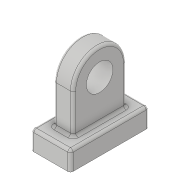
# Autodesk Inventor part: Pivot
Saved by Autodesk Inventor 2017 (Build 210142000, 142)
## iProperties
Created: 2016-07-28
Part Number: Pivot
Material: Generic
Document SubType Name: Modeling
Designer: Tutorial Books
Density: 1 g/cm^3
Appearance: Default
Author: Tutorial Books
Autodesk Inventor part; units mm, degrees
ref_plane "YZ Plane" through (0, 0, 0) normal (1, 0, 0) x (0, 1, 0)
ref_plane "XZ Plane" through (0, 0, 0) normal (0, 1, 0) x (-1, 0, 0)
ref_plane "XY Plane" through (0, 0, 0) normal (0, 0, 1) x (1, 0, 0)
sketch "Sketch1" plane through (0, 0, 0) normal (0, 1, 0) x (-1, 0, 0)
  line L0 (7.493, 14.986) -> (-7.493, 14.986)
  line L1 (-7.493, 14.986) -> (-7.493, -14.986)
  line L2 (-7.493, -14.986) -> (7.493, -14.986)
  line L3 (7.493, -14.986) -> (7.493, 14.986)
  line L4 (7.493, 14.986) -> (-7.493, -14.986) construction
  line L5 (-7.493, 14.986) -> (7.493, -14.986) construction
  point P0 (0, 0)
  dimension "d0" = 29.972
  dimension "d1" = 14.986
  constraints: 12 end point, 2 midpoint, 2 parallel, 1 horizontal, 1 perpendicular
  measures "d0" distance of L0.end L1.end
  measures "d1" distance of L1.end L2.end
extrude "Extrusion1" add sketch "Sketch1" along normal blind 7.366
sketch "Sketch2" plane through (0, 0, 0) normal (1, 0, 0) x (0, 1, 0)
  line L0 (7.366, 14.986) -> (7.366, -14.986) projected
  line L1 (7.366, 10.16) -> (22.352, 10.16)
  arc A0 (22.352, -10.16) -> (22.352, 10.16) centre (22.352, 0) ccw
  line L2 (22.352, -10.16) -> (7.366, -10.16)
  line L3 (7.366, 10.16) -> (7.366, -10.16)
  circle A1 centre (22.352, 0) radius 5.08
  point P0 (0, 0)
  dimension "d4" = 14.986
  dimension "d5" = 10.16
  dimension "d6" = 10.16
  dimension "d7" = 10.16
  constraints: 6 end point, 2 centre point, 2 point on circle, 2 point on line, 2 tangent, 1 coincident, 1 collinear, 1 horizontal, 1 parallel
  measures "d4" distance from line of L0 A0.centre
  measures "d5" radius of A0
  measures "d6" diameter of A1
  measures "d7" distance from line of L1 point (0, 0)
extrude "Extrusion2" add sketch "Sketch2" along normal mid plane 7.366
fillet "Fillet1" radius 1.016 7 edges at (7.493, 3.683, 14.986) (7.493, 7.366, 0) (7.493, 3.683, -14.986) (0, 7.366, -14.986) (0, 7.366, 14.986) (-7.493, 3.683, 14.986) (-7.493, 7.366, 0)
fillet "Fillet2" radius 1.016 6 edges at (3.683, 32.512, 0) (3.683, 14.859, -10.16) (3.683, 14.859, 10.16) (-3.683, 32.512, 0) (-3.683, 14.859, -10.16) (-3.683, 14.859, 10.16)
fillet "Fillet3" radius 1.016 8 edges at (3.3854, 7.366, 9.8624) (0, 7.366, 10.16) (-3.3854, 7.366, 9.8624) (-3.683, 7.366, 0) (-3.3854, 7.366, -9.8624) (0, 7.366, -10.16) (3.3854, 7.366, -9.8624) (3.683, 7.366, 0)
fillet "Fillet4" radius 1.016 2 edges at (-7.1954, 7.0684, -14.6884) (-7.493, 3.175, -14.986)
body "Solid1"
